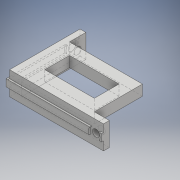
# Autodesk Inventor part: SuporteRJ45
Saved by Autodesk Inventor 2017 (Build 210142000, 142)
## iProperties
Created: 2020-11-22
Part Number: SuporteRJ45
Material: Generic
Document SubType Name: Modeling
Designer: ale
Density: 1 g/cm^3
Appearance: Default
Author: ale
Autodesk Inventor part; units mm, degrees
ref_plane "YZ Plane" through (0, 0, 0) normal (1, 0, 0) x (0, 1, 0)
ref_plane "XZ Plane" through (0, 0, 0) normal (0, 1, 0) x (-1, 0, 0)
ref_plane "XY Plane" through (0, 0, 0) normal (0, 0, 1) x (1, 0, 0)
sketch "Sketch1" plane through (0, 0, 0) normal (0, 0, 1) x (1, 0, 0)
  line L0 (-21.1, 10.5) -> (21.1, 10.5)
  line L1 (21.1, 10.5) -> (21.1, -10.5)
  line L2 (21.1, -10.5) -> (-21.1, -10.5)
  line L3 (-21.1, -10.5) -> (-21.1, 10.5)
  line L4 (-21.1, 10.5) -> (21.1, -10.5) construction
  line L5 (21.1, 10.5) -> (-21.1, -10.5) construction
  line L6 (31.1, 20.5) -> (-31.1, 20.5)
  line L7 (-31.1, 20.5) -> (-31.1, -20.5)
  line L8 (-31.1, -20.5) -> (31.1, -20.5)
  line L9 (31.1, -20.5) -> (31.1, 20.5)
  point P0 (0, 0)
  dimension "d0" = 42.2
  dimension "d1" = 21
  dimension "d2" = 10
  constraints: 20 end point, 4 parallel, 2 midpoint, 2 perpendicular, 1 horizontal, 3 other
  measures "d0" distance of L1.end L2.end
  measures "d1" distance of L0.end L1.end
  measures "d2" distance between parallel lines of L0 L6
extrude "Extrusion1" add sketch "Sketch1" along normal blind 9
sketch "Sketch2" plane through (-31.1, -20.5, 0) normal (0, -1, 0) x (1, 0, 0)
  line L0 (62.2, 9) -> (0, 9) projected
  line L1 (0, 9) -> (75, 9)
  line L2 (75, 9) -> (75, -11)
  line L3 (75, -11) -> (0, -11)
  line L4 (0, -11) -> (0, 9)
  point P0 (31.1, 0)
  dimension "d5" = 75
  dimension "d6" = 20
  constraints: 8 end point, 2 parallel, 1 horizontal, 1 perpendicular
  measures "d5" distance of L2.end L3.end
  measures "d6" distance of L1.end L2.end
extrude "Extrusion2" add sketch "Sketch2" along normal blind 5
sketch "Sketch3" plane through (-31.1, 20.5, 0) normal (-1, 0, 0) x (0, 0, 1)
  line L0 (9, -46) -> (-11, -46) projected
  line L1 (9, -46) -> (-11, -46)
  line L2 (-11, -46) -> (-11, 14)
  line L3 (-11, 14) -> (9, 14)
  line L4 (9, 14) -> (9, -46)
  point P0 (0, -20.5)
  dimension "d9" = 20
  dimension "d10" = 60
  constraints: 8 end point, 2 parallel, 1 horizontal, 1 perpendicular
  measures "d9" distance of L2.end L3.end
  measures "d10" distance of L1.end L2.end
extrude "Extrusion3" add sketch "Sketch3" along normal blind 5
sketch "Sketch4" plane through (-31.1, -25.5, 0) normal (0, -1, 0) x (1, 0, 0)
  line L0 (75, 9) -> (75, -11) projected
  line L1 (75, 2.3333) -> (-5, 2.3333)
  line L2 (-5, -11) -> (-5, 9) projected
  line L3 (75, -3.6667) -> (-5, -3.6667)
  line L4 (75, 9) -> (-5, 9) projected
  line L5 (75, 2.3333) -> (75, -3.6667)
  line L6 (-5, 2.3333) -> (-5, -3.6667)
  point P0 (31.1, 0)
  dimension "d13" = 6
  dimension "d14" = 6.6667
  constraints: 8 end point, 2 perpendicular, 2 point on line, 1 horizontal, 1 parallel
  measures "d13" distance between parallel lines of L1 L3
  measures "d14" distance between parallel lines of L1 L4
extrude "Extrusion4" add sketch "Sketch4" along normal blind 1.5 contours L0 L3 L2 L1
sketch "Sketch5" plane through (-36.1, 20.5, 0) normal (-1, 0, 0) x (0, 0, 1)
  line L0 (2.353, -47.5) -> (2.353, 14)
  line L1 (9, 14) -> (-11, 14) projected
  line L2 (2.3333, -47.5) -> (-3.6667, -47.5) projected
  line L3 (-3.6667, -47.5) -> (-3.6667, 14)
  line L4 (-3.6667, 14) -> (2.353, 14)
  line L5 (2.353, -47.5) -> (-3.6667, -47.5)
  point P0 (0, -20.5)
  constraints: 8 end point, 2 vertical, 1 horizontal, 1 perpendicular, 1 point on line
extrude "Extrusion5" add sketch "Sketch5" along normal blind 1.5
sketch "Sketch6" plane through (-37.6, 20.5, 0) normal (-1, 0, 0) x (0, 0, 1)
  line L0 (9, 14) -> (2.353, 14) projected
  line L1 (0, 0) -> (9, 0) projected
  line L2 (9, -46) -> (9, 14) projected
  line L3 (-11, 14) -> (-11, -46) projected
  point P0 (0, -20.5)
  point P1 (-1, 7)
  dimension "d19" = 14
  dimension "d20" = 20
  dimension "d21" = 10
  dimension "d22" = 7
  measures "d19" distance between parallel lines of L0 L1
  measures "d20" distance between parallel lines of L2 L3
  measures "d21" distance from line of L3 point (-1, 7)
  measures "d22" distance from line of L0 point (-1, 7)
hole "Hole1" at (-37.6, 27.5, -1) direction (1, 0, 0) diameter 6 end through all counterbore diameter 10 counterbore depth 1.5
sketch "Sketch7" plane through (-31.1, -27, 0) normal (0, -1, 0) x (1, 0, 0)
  line L0 (75, 2.3333) -> (75, 9) projected
  line L1 (62.2, 0) -> (62.2, 9) projected
  line L2 (75, -11) -> (-5, -11) projected
  line L3 (75, 9) -> (-5, 9) projected
  point P0 (31.1, 0)
  point P1 (68.6, -1)
  dimension "d30" = 12.8
  dimension "d31" = 20
  dimension "d32" = 10
  dimension "d33" = 6.4
  measures "d30" distance between parallel lines of L0 L1
  measures "d31" distance between parallel lines of L2 L3
  measures "d32" distance from line of L3 point (68.6, -1)
  measures "d33" distance from line of L0 point (68.6, -1)
hole "Hole2" at (37.5, -27, -1) direction (0, 1, 0) diameter 6 end through all counterbore diameter 10 counterbore depth 1.5
equation "\"d21\" = 0.5 * d20"
equation "\"d22\" = 0.5 * d19"
equation "\"d32\" = 0.5 * d31"
equation "\"d33\" = 0.5 * d30"
body "Solid1"
